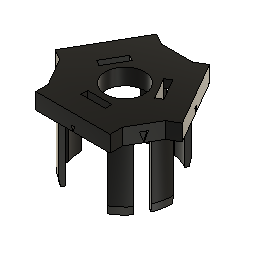
LASER_CUTTER_JIG v8 (Autodesk Fusion 360 design; units mm, degrees)
Autodesk Fusion 360 part; units mm, degrees
note: some values were not read from the file. Chosen so that the rebuilt part matches the saved one: which face or edge a step refers to; which pieces of a blend or face edit are solid.
sketch "Sketch1" plane through (0, 0, 0) normal (0, 0, 1) x (1, 0, 0)
  circle A0 centre (0, 0) radius 30
  circle A1 centre (0, 0) radius 32
  line L0 (39.1562, -3.8206) -> (16.2694, 35.8206)
  line L1 (-16.2694, 35.8206) -> (-39.1562, -3.8206)
  line L2 (-22.8868, -32) -> (22.8868, -32)
  line L3 (-22.8868, -32) -> (-22.8868, -24.3588)
  line L4 (-27.7128, -16) -> (-22.8868, -24.3588)
  line L5 (-39.1562, -3.8206) -> (-32.5388, -7.6412)
  line L6 (-27.7128, -16) -> (-32.5388, -7.6412)
  line L7 (39.1562, -3.8206) -> (32.5388, -7.6412)
  line L8 (27.7128, -16) -> (22.8868, -24.3588)
  line L9 (22.8868, -32) -> (22.8868, -24.3588)
  line L10 (27.7128, -16) -> (32.5388, -7.6412)
  line L11 (-16.2694, 35.8206) -> (-9.652, 32)
  line L12 (0, 32) -> (9.652, 32)
  line L13 (16.2694, 35.8206) -> (9.652, 32)
  line L14 (0, 32) -> (-9.652, 32)
  line L15 (-4, 29.7321) -> (-4, 26.7021)
  line L16 (-13.5, 23.3827) -> (-15, 25.9808)
  line L17 (0, 0) -> (30, 0) construction
  arc A2 (-4, 26.7021) -> (-13.5, 23.3827) centre (0, 0) ccw
  line L18 (4, 29.7321) -> (4, 26.7021)
  arc A3 (13.5, 23.3827) -> (4, 26.7021) centre (0, 0) ccw
  line L19 (13.5, 23.3827) -> (15, 25.9808)
  line L20 (-27, 0) -> (-30, 0)
  arc A4 (-27, 0) -> (-25.1247, -9.8869) centre (0, 0) ccw
  line L21 (-27.7488, -11.402) -> (-25.1247, -9.8869)
  line L22 (-23.7488, -18.3302) -> (-21.1247, -16.8151)
  line L23 (-13.5, -23.3827) -> (-15, -25.9808)
  arc A5 (-21.1247, -16.8151) -> (-13.5, -23.3827) centre (0, 0) ccw
  line L24 (13.5, -23.3827) -> (15, -25.9808)
  arc A6 (13.5, -23.3827) -> (21.1247, -16.8151) centre (0, 0) ccw
  line L25 (23.7488, -18.3302) -> (21.1247, -16.8151)
  line L26 (27.7488, -11.402) -> (25.1247, -9.8869)
  line L27 (27, 0) -> (30, 0)
  arc A7 (25.1247, -9.8869) -> (27, 0) centre (0, 0) ccw
  line L28 (7.5, -15.4872) -> (-7.5, -15.4872)
  line L29 (-7.5, -15.4872) -> (-7.5, -19.5872)
  line L30 (-7.5, -19.5872) -> (7.5, -19.5872)
  line L31 (7.5, -19.5872) -> (7.5, -15.4872)
  line L32 (20.713, 3.2984) -> (13.213, 16.2888)
  line L33 (13.213, 16.2888) -> (9.6623, 14.2388)
  line L34 (9.6623, 14.2388) -> (17.1623, 1.2484)
  line L35 (17.1623, 1.2484) -> (20.713, 3.2984)
  line L36 (-13.213, 16.2888) -> (-20.713, 3.2984)
  line L37 (-20.713, 3.2984) -> (-17.1623, 1.2484)
  line L38 (-17.1623, 1.2484) -> (-9.6623, 14.2388)
  line L39 (-9.6623, 14.2388) -> (-13.213, 16.2888)
  circle A8 centre (0, 0) radius 12
  line L40 (0, 0) -> (0, -15.4872) construction
  dimension "d1" = 60
  dimension "d77" = 64
  dimension "d79" = 360
  dimension "d80" = 120
  dimension "d82" = 360
  dimension "d84" = 360
  dimension "d85" = 4.1
  dimension "d116" = 15
  constraint coincident A0.centre A1.centre
  constraint perpendicular L2 L3
  constraint tangent A1 L4
  constraint vertical L15
  constraint horizontal L17
  constraint coincident A0 L16.end
  constraint coincident A0 L15.start
  constraint horizontal L28
  constraint vertical L29
  constraint horizontal L30
  constraint vertical L31
  constraint concentric A7 A8
  constraint midpoint L28 L40.end
  constraint perpendicular L28 L40
  measures "d1" diameter of A0
  measures "d77" diameter of A1
  measures "d80" angle of L16 L17
  measures "d85" distance of L28 L30
  measures "d116" distance of L29.end L30.end
extrude "Extrude10" add sketch "Sketch1" along normal blind 10 contours A0 L15 L16 A2 L18 A3 L19 L20 A4 L21 L22 L23 A5 L24 A6 L25 L26 L27 A7 | A0 L26 L27 A7 | A0 L18 A3 L19 | A0 L24 A6 L25 | A0 L15 L16 A2 | A0 L22 L23 A5 | A0 L20 A4 L21 | A1 | A1 L2 L8 L9 | A1 L0 L7 L10 | A1 L2 L3 L4 | A1 L0 L12 L13 | A1 L1 L5 L6 | A1 L1 L11 L14 | A8
extrude "Extrude11" add sketch "Sketch1" against normal blind 40 contours A0 L26 L27 A7 | A0 L18 A3 L19 | A0 L24 A6 L25 | A0 L15 L16 A2 | A0 L22 L23 A5 | A0 L20 A4 L21
chamfer "Chamfer5" distance 1 distance2 5 6 edges at (-19.7484, -22.5832, -40) (-29.4318, -5.811, -40) (-9.6834, 28.3942, -40) (9.6834, 28.3942, -40) (29.4318, -5.811, -40) (19.7484, -22.5832, -40) measured on face at (-22.0155, -18.7995, -40) measured on face at (-27.2886, -9.6662, -40) measured on face at (-5.2731, 28.4658, -40) measured on face at (5.2731, 28.4658, -40) measured on face at (27.2886, -9.6662, -40) measured on face at (22.0155, -18.7995, -40)
extrude "Extrude12" cut sketch "Sketch1" along normal blind 10 contours A8
sketch "Sketch10" plane through (27.7128, 16, 0) normal (0.866025, 0.5, 0) x (-0.5, 0.866025, 0)
  line L0 (-22.8868, 0) -> (22.8868, 0)
  line L1 (22.8868, 0) -> (22.8868, 10)
  line L2 (22.8868, 10) -> (-22.8868, 10)
  line L3 (-22.8868, 10) -> (-22.8868, 0)
  line L4 (0, 0) -> (-2, 6)
  line L5 (-2, 6) -> (0, 6)
  line L6 (0, 6) -> (0, 0) construction
  line L7 (0, 0) -> (2, 6)
  line L8 (2, 6) -> (0, 6)
  constraint coincident L4.start L6.end
  constraint parallel L0 L5
  constraint perpendicular L0 L6
  constraint symmetric L4.start L6 L7.start
  constraint symmetric L4.end L6 L7.end
  constraint symmetric L5.end L6 L8.end
extrude "Extrude13" cut sketch "Sketch10" against normal blind 1 contours L4 L5 L7 L8
fillet "Fillet6" radius 0.75 1 edges at (26.8468, 15.5, 6)
pattern_circular "C-Pattern5" count 6 over 360 about axis through (0, 0, 1.75) along (0, 0, 1) of "Extrude13", "Fillet6"
sketch "Sketch11" plane through (0, 0, 0) normal (0, 0, 1) x (1, 0, 0)
  circle A0 centre (0, 0) radius 14.4222
  circle A1 centre (0, 0) radius 27
  line L0 (7.1162, -12.5443) -> (7.1162, -26.0453)
  line L1 (7.1162, -21.8938) -> (0, -21.8938)
  line L2 (0, 1.75) -> (0, 22.5)
  line L3 (-7.1162, -12.5443) -> (-7.1162, -26.0453)
  line L4 (-7.1162, -21.8938) -> (0, -21.8938)
  line L5 (15.4025, 17.1097) -> (18.9606, 10.9469)
  line L6 (7.3056, 12.435) -> (18.9978, 19.1855)
  line L7 (14.4218, 0.1093) -> (26.114, 6.8599)
  line L8 (22.5187, 4.7841) -> (18.9606, 10.9469)
  line L9 (-22.5187, 4.7841) -> (-18.9606, 10.9469)
  line L10 (-14.4218, 0.1093) -> (-26.114, 6.8599)
  line L11 (-7.3056, 12.435) -> (-18.9978, 19.1855)
  line L12 (-15.4025, 17.1097) -> (-18.9606, 10.9469)
  arc A2 (13.5, -23.3827) -> (21.1247, -16.8151) centre (0, 0) ccw
  dimension "d101" = 360
  constraint coincident A0.centre A1.centre
  constraint concentric A0 A1
  constraint coincident A0 L0.start
  constraint coincident A1 L0.end
  constraint vertical L0
  constraint coincident L0 L1.start
  constraint perpendicular L0 L1
  constraint symmetric L0.start L2 L3.start
  constraint symmetric L0.end L2 L3.end
  constraint symmetric L1.start L2 L4.start
  constraint symmetric L1.end L2 L4.end
  constraint tangent A1 A2
extrude "Extrude14" cut sketch "Sketch11" along normal blind 5 contours A0 A1 L0 L7 A2 | A0 A1 L6 L11 | A1 L5 L6 L7 L8 | A0 A1 L3 L10 | A1 L0 L1 L3 L4 | A1 L9 L10 L11 L12
delete_face "DeleteFace1" 1 faces at (27.2278, 15.0096, 5.5963)
extrude "Extrude15" add 1 faces at (26.8468, 15.5, 4) along direction (0.866025, 0.5, 0) blind 1
delete_face "DeleteFace2" 1 faces at (-0.6152, -31.0847, 5.5963)
extrude "Extrude16" add 1 faces at (0, -31, 4) along direction (0, -1, 0) blind 1
delete_face "DeleteFace3" 1 faces at (-27.2278, 15.0096, 5.5963)
extrude "Extrude17" add 1 faces at (-26.8468, 15.5, 4) along direction (-0.866025, 0.5, 0) blind 1
sketch "Sketch12" plane through (0, -32, 0) normal (0, -1, 0) x (1, 0, 0)
  line L0 (-22.8868, 0) -> (22.8868, 0)
  line L1 (22.8868, 0) -> (22.8868, 10)
  line L2 (22.8868, 10) -> (-22.8868, 10)
  line L3 (-22.8868, 10) -> (-22.8868, 0)
  line L4 (0, 0) -> (-1, 3)
  line L5 (-1, 3) -> (0, 3)
  line L6 (0, 3) -> (0, 0) construction
  line L7 (0, 0) -> (1, 3)
  line L8 (1, 3) -> (0, 3)
  constraint coincident L4.start L6.end
  constraint parallel L0 L5
  constraint perpendicular L0 L6
  constraint symmetric L4.start L6 L7.start
  constraint symmetric L4.end L6 L7.end
  constraint symmetric L5.end L6 L8.end
extrude "Extrude18" cut sketch "Sketch12" against normal blind 1.6 contours L4 L5 L7 L8
fillet "Fillet7" radius 1.55 tangency weight 1.08583 4 edges at (1, -31.2, 3) (0.5, -30.4, 3) (-1, -31.2, 3) (-0.5, -30.4, 3)
pattern_circular "C-Pattern6" count 3 over 360 about axis through (0, 0, 1.75) along (0, 0, 1) of "Extrude18", "Fillet7"
equation "d77 = 60 mm + 4 mm"
